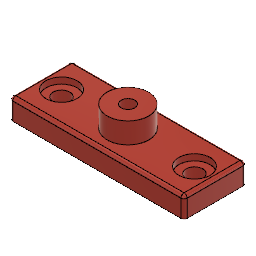
Y-belt-tensioner-III-rev1 v20 v3 (Autodesk Fusion 360 design; units mm, degrees)
Autodesk Fusion 360 part; units mm, degrees
sketch "Sketch1" plane through (0, 0, 0) normal (0, 1, 0) x (1, 0, 0)
  line L0 (21, -7.5) -> (-21, -7.5)
  line L1 (-21, -7.5) -> (-21, 7.5)
  line L2 (-21, 7.5) -> (21, 7.5)
  line L3 (21, 7.5) -> (21, -7.5)
  dimension "d1" = 42
  dimension "d2" = 15
  dimension "d3" = 7.5
  dimension "d4" = 21
  measures "d3" distance of origin L2
  measures "d4" distance of origin L1
extrude "Extrude1" add sketch "Sketch1" along normal blind 5
sketch "Sketch2" plane through (0, 5, 0) normal (0, 1, 0) x (-1, 0, 0)
  line L0 (-21, -7.5) -> (21, -7.5)
  line L1 (21, -7.5) -> (21, 7.5)
  line L2 (21, 7.5) -> (-21, 7.5)
  line L3 (-21, 7.5) -> (-21, -7.5)
  circle A0 centre (0, 0) radius 5
  dimension "d7" = 10
  measures "d7" diameter of A0
extrude "Extrude2" add sketch "Sketch2" along normal blind 5 contours A0
sketch "Sketch3" plane through (0, 10, 0) normal (0, 1, 0) x (-1, 0, 0)
  circle A0 centre (0, 0) radius 5
  circle A1 centre (0, 0) radius 1.625
  dimension "d10" = 3.25
  measures "d10" diameter of A1
extrude "Extrude6" cut sketch "Sketch3" against normal blind 7.5 contours A1
sketch "Sketch7" plane through (0, 5, 0) normal (0, 1, 0) x (-1, 0, 0)
  circle A0 centre (0, 0) radius 5
  line L0 (-21, -7.5) -> (21, -7.5)
  line L1 (21, -7.5) -> (21, 7.5)
  line L2 (21, 7.5) -> (-21, 7.5)
  line L3 (-21, 7.5) -> (-21, -7.5)
  circle A1 centre (16, 0.0057) radius 2
  circle A2 centre (-16, 0.0028) radius 2
  dimension "d23" = 32
  dimension "d24" = 16
  dimension "d25" = 4
  dimension "d26" = 4
  measures "d24" distance of A0.centre
  measures "d25" diameter of A1
  measures "d26" diameter of A2
extrude "Extrude7" cut sketch "Sketch7" against normal through all contours A1 | A2
fillet "Fillet1" radius 0.75 8 edges at (0, 5, -7.5) (-21, 5, 0) (21, 5, 0) (0, 5, 7.5) (-21, 2.5, 7.5) (21, 2.5, 7.5) (21, 2.5, -7.5) (-21, 2.5, -7.5)
sketch "Sketch8" plane through (0, 5, 0) normal (0, 1, 0) x (-1, 0, 0)
  circle A0 centre (16, 0.0057) radius 2
  circle A1 centre (-16, 0.0028) radius 2
  circle A2 centre (16, 0.0057) radius 3.75
  circle A3 centre (-16, 0.0028) radius 3.75
  dimension "d29" = 7.5
  dimension "d30" = 7.5
  measures "d29" diameter of A2
  measures "d30" diameter of A3
extrude "Extrude8" cut sketch "Sketch8" against normal blind 1.5
